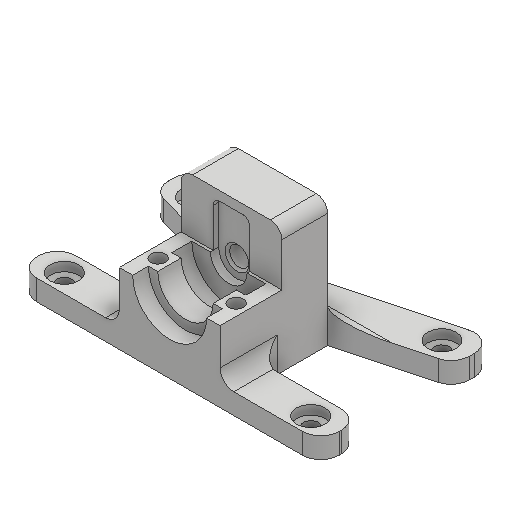
# Autodesk Inventor part: 3DP_ABS_E3DV6_Mount
Saved by Autodesk Inventor 2026.1 (Build 301233000, 233)
## iProperties
Created: 2016-01-25
Part Number: 3DP_ABS_E3DV6_Mount
Material: Ogólny
Document SubType Name: Modeling
Designer: Andrzej
Density: 1 g/cm^3
Appearance: Domyślna
Mass: 12.8574 g
Surface Area: 66.9041 cm^2
Volume: 12.8574 cm^3
Author: Andrzej
Autodesk Inventor part; units mm, degrees
ref_plane "YZ Plane" through (0, 0, 0) normal (1, 0, 0) x (0, 1, 0)
ref_plane "XZ Plane" through (0, 0, 0) normal (0, 1, 0) x (-1, 0, 0)
ref_plane "XY Plane" through (0, 0, 0) normal (0, 0, 1) x (1, 0, 0)
sketch "Szkic1" plane through (0, 0, 0) normal (0, 0, 1) x (1, 0, 0)
  line L0 (-43.0447, 20.476) -> (-43.0447, -18.4903)
  line L1 (22.9553, 20.2216) -> (22.9553, -18.4903)
  line L2 (-21.0447, 5.0097) -> (-21.0447, -9.9903)
  line L3 (0.9553, 5.0097) -> (0.9553, -9.9903)
  line L4 (-43.0447, -18.4903) -> (22.9553, -18.4903)
  line L5 (-43.0447, -9.9903) -> (-21.0447, -9.9903)
  line L6 (0.9553, -9.9903) -> (22.9553, -9.9903)
  line L7 (-21.0447, 5.0097) -> (0.9553, 5.0097)
  line L8 (-21.0447, 5.0097) -> (-43.0447, 11.1338)
  line L9 (-10.2095, 11.3357) -> (-43.0447, 20.476)
  line L10 (0.9553, 5.0097) -> (22.9553, 10.9042)
  line L11 (-10.2095, 11.3357) -> (22.9553, 20.2216)
  point P0 (0, 0)
  point P1 (-37.0447, -14.4903)
  point P2 (16.955, -14.6697)
  point P3 (-37.0447, 14.1347)
  point P4 (16.9553, 13.9553)
  dimension "d0" = 66
  dimension "d1" = 54
  dimension "d2" = 6
  dimension "d3" = 54
  dimension "d4" = 6
  dimension "d5" = 28.625
  dimension "d6" = 22
  dimension "d7" = 22
  dimension "d8" = 4
  dimension "d10" = 23.5
  dimension "d11" = 4.5
  dimension "d12" = 9
  dimension "d13" = 28.625
  dimension "d14" = 4.5
  dimension "d15" = 9
  constraints: 24 end point, 4 perpendicular, 4 point on line, 4 vertical
  measures "d0" distance between parallel lines of L1 L0
  measures "d1" distance of point (16.955, -14.67) point (-37.045, -14.49)
  measures "d2" distance from line of L0 point (-37.045, -14.49)
  measures "d3" horizontal distance of point (16.955, 13.955) point (-37.045, 14.135)
  measures "d4" distance from line of L0 point (-37.045, 14.135)
  measures "d5" distance of point (-37.045, -14.49) point (-37.045, 14.135)
  measures "d6" distance between parallel lines of L3 L2
  measures "d7" distance between parallel lines of L2 L0
  measures "d8" distance from line of L4 point (-37.045, -14.49)
  measures "d10" distance between parallel lines of L4 L7
  measures "d11" distance from line of L8 point (-37.045, 14.135)
  measures "d12" distance between parallel lines of L8 L9
  measures "d13" distance of point (16.955, -14.67) point (16.955, 13.955)
  measures "d14" distance from line of L10 point (16.955, 13.955)
  measures "d15" distance between parallel lines of L10 L11
extrude "Wyciągnięcie proste1" add sketch "Szkic1" along normal blind 4.5 contours L9 L11 L1 L10 L7 L8 L0 | L5 L2 L7 L3 L6 L1 L4 L0
hole "Otwór1" at (-37.0447, -14.4903, 0) at (16.955, -14.6697, 0) at (-37.0447, 14.1347, 0) at (16.9553, 13.9553, 0) direction (0, 0, 1) diameter 3.25 end through all
sketch "Szkic2" plane through (0, 0, 4.5) normal (0, 0, 1) x (1, 0, 0)
  line L0 (-21.0447, 5.0097) -> (-21.0447, -9.9903) projected
  line L1 (-21.0447, 5.0097) -> (0.7211, 5.0097)
  circle A0 centre (-37.0447, 14.1347) radius 1.625 projected
  circle A1 centre (-37.0447, -14.4903) radius 1.625 projected
  circle A2 centre (16.955, -14.6697) radius 1.625 projected
  circle A3 centre (16.9553, 13.9553) radius 1.625 projected
  line L2 (-43.0447, 20.476) -> (-43.0447, 11.1338) projected
  line L3 (-43.0447, 11.1338) -> (-21.0447, 5.0097) projected
  line L4 (-21.0447, 5.0097) -> (-21.0447, -9.9903) projected
  line L5 (-21.0447, -9.9903) -> (-43.0447, -9.9903) projected
  line L6 (-43.0447, -9.9903) -> (-43.0447, -18.4903) projected
  line L7 (-43.0447, -18.4903) -> (22.9553, -18.4903) projected
  line L8 (22.9553, -18.4903) -> (22.9553, -9.9903) projected
  line L9 (22.9553, -9.9903) -> (0.9553, -9.9903) projected
  line L10 (0.9553, -9.9903) -> (0.9553, 5.0097) projected
  line L11 (0.9553, 5.0097) -> (22.9553, 10.9042) projected
  line L12 (22.9553, 10.9042) -> (22.9553, 20.2216) projected
  line L13 (22.9553, 20.2216) -> (-10.2095, 11.3357) projected
  line L14 (-10.2095, 11.3357) -> (-43.0447, 20.476) projected
  line L15 (-21.0447, -4.9903) -> (0.9553, -4.9903)
  line L16 (-43.0447, -18.4903) -> (22.9553, -18.4903) projected
  line L17 (-21.0447, -4.9903) -> (0.9553, -4.9903)
  line L18 (0.9553, -4.9903) -> (0.9553, -18.4903)
  line L19 (0.9553, -18.4903) -> (-21.0447, -18.4903)
  line L20 (-21.0447, -18.4903) -> (-21.0447, -4.9903)
  line L21 (-21.0447, 5.0097) -> (0.9553, 5.0097)
  line L22 (0.9553, 5.0097) -> (0.9553, -4.9903)
  line L23 (0.9553, -4.9903) -> (-21.0447, -4.9903)
  line L24 (-21.0447, -4.9903) -> (-21.0447, 5.0097)
  circle A4 centre (-37.0447, 14.1347) radius 3.1
  circle A5 centre (16.9553, 13.9553) radius 3.1
  circle A6 centre (16.955, -14.6697) radius 3.1
  circle A7 centre (-37.0447, -14.4903) radius 3.1
  point P0 (0, 0)
  dimension "d25" = 13.5
  dimension "d31" = 6.2
  dimension "d32" = 6.2
  dimension "d33" = 6.2
  dimension "d34" = 6.2
  constraints: 20 end point, 4 centre point, 4 coincident, 4 parallel, 3 horizontal, 3 perpendicular, 3 point on line
  measures "d25" distance between parallel lines of L7 L15
  measures "d31" diameter of A4
  measures "d32" diameter of A5
  measures "d33" diameter of A6
  measures "d34" diameter of A7
extrude "Wyciągnięcie proste2" add sketch "Szkic2" along normal blind 11 contours L15 L10 L18 L7 L20 L0
extrude "Wyciągnięcie proste3" add sketch "Szkic2" along normal blind 23 contours L1 L21 L10 L15 L0
fillet "Zaokrąglenie1" radius 4 11 edges at (22.9553, 10.9042, 2.25) (22.9553, 20.2216, 2.25) (-10.2095, 11.3357, 2.25) (-43.0447, 20.476, 2.25) (-43.0447, 11.1338, 2.25) (0.9553, -9.9903, 2.25) (22.9553, -9.9903, 2.25) (22.9553, -18.4903, 2.25) (-43.0447, -18.4903, 2.25) (-43.0447, -9.9903, 2.25) (-21.0447, -9.9903, 2.25)
extrude "Wyciągnięcie proste4" cut sketch "Szkic2" against normal blind 2 contours A4 | A5 | A6 | A7
fillet "Zaokrąglenie2" radius 3 3 edges at (-10.0447, 5.0097, 4.5) (-21.0447, -12.2403, 4.5) (0.9553, -12.2403, 4.5)
fillet "Zaokrąglenie3" radius 2.5 2 edges at (-21.0447, 0.0097, 27.5) (0.9553, 0.0097, 27.5)
sketch "Szkic3" plane through (-21.0447, -18.4903, 15.5) normal (0, -1, 0) x (1, 0, 0)
  line L0 (22, 0) -> (0, 0) projected
  line L1 (0, -8) -> (0, 0) projected
  arc A0 (2.925, 0) -> (19.075, 0) centre (11, 0) ccw
  arc A1 (4.95, 0) -> (17.05, 0) centre (11, 0) ccw
  point P0 (21.0447, -15.5)
  dimension "d39" = 11
  dimension "d48" = 16.15
  dimension "d51" = 12.1
  constraints: 4 point on circle, 4 point on line, 2 centre point, 2 coincident, 1 midpoint
  measures "d39" distance from line of L1 point (11, 0)
  measures "d48" diameter of A0
  measures "d51" diameter of A1
hole "Otwór2" at (-10.0447, -18.4903, 15.5) direction (0, 1, 0) diameter 4.2 end through all
extrude "Wyciągnięcie proste5" cut sketch "Szkic3" against normal blind 12.9
extrude "Wyciągnięcie proste6" add sketch "Szkic3" against normal blind 8.55 contours A0 L0 A1
extrude "Wyciągnięcie proste7" cut sketch "Szkic3" against normal blind 3.45 contours A0 L0 A1
sketch "Szkic4" plane through (0, 0, 15.5) normal (0, 0, 1) x (1, 0, 0)
  line L0 (-3.9947, -15.0403) -> (-1.9697, -15.0403) projected
  line L1 (-3.9947, -9.9403) -> (-1.9697, -9.9403) projected
  line L2 (0.9553, -18.4903) -> (0.9553, -4.9903) projected
  line L3 (-3.9947, -15.0403) -> (-3.9947, -9.9403) projected
  line L4 (-18.1197, -9.9403) -> (-16.0947, -9.9403) projected
  line L5 (-21.0447, -4.9903) -> (-21.0447, -18.4903) projected
  point P0 (0, 0)
  point P1 (-18.5697, -12.4903)
  point P2 (-1.5197, -12.4903)
  dimension "d56" = 5.1
  dimension "d57" = 4.95
  dimension "d58" = 2.475
  dimension "d59" = 2.55
  dimension "d60" = 2.55
  dimension "d61" = 2.475
  measures "d56" distance between parallel lines of L0 L1
  measures "d57" distance between parallel lines of L2 L3
  measures "d58" distance from line of L2 point (-1.52, -12.49)
  measures "d59" distance from line of L1 point (-1.52, -12.49)
  measures "d60" distance from line of point (-18.57, -12.49) L4
  measures "d61" distance from line of point (-18.57, -12.49) L5
hole "Otwór3" at (-18.5697, -12.4903, 15.5) at (-1.5197, -12.4903, 15.5) direction (0, 0, -1) diameter 3.2 end through all
sketch "Szkic5" plane through (0, 0, 0) normal (0, 0, -1) x (-1, 0, 0)
  circle A0 centre (18.5697, -12.4903) radius 1.6 projected
  circle A1 centre (1.5197, -12.4903) radius 1.6 projected
  circle A2 centre (18.5697, -12.4903) radius 3.1
  circle A3 centre (1.5197, -12.4903) radius 3.1
  point P0 (0, 0)
  dimension "d69" = 6.2
  dimension "d70" = 6.2
  constraints: 2 centre point, 2 coincident
  measures "d69" diameter of A2
  measures "d70" diameter of A3
extrude "Wyciągnięcie proste8" cut sketch "Szkic5" against normal blind 3
sketch "Szkic6" plane through (-21.0447, -5.5903, 15.5) normal (0, -1, 0) x (1, 0, 0)
  arc A0 (7, 0) -> (15, 0) centre (11, 0) ccw
  line L0 (7, 0) -> (7, 8.5)
  line L1 (8.5, 10) -> (13.5, 10)
  line L2 (15, 8.5) -> (15, 0)
  arc A1 (8.9, 0) -> (13.1, 0) centre (11, 0) ccw projected
  arc A2 (8.5, 10) -> (7, 8.5) centre (8.5, 8.5) ccw
  arc A3 (15, 8.5) -> (13.5, 10) centre (13.5, 8.5) ccw
  point P0 (21.0447, -15.5)
  point P1 (7, 10)
  dimension "d73" = 8
  dimension "d74" = 10
  dimension "d75" = 1.5
  constraints: 6 end point, 6 point on circle, 5 tangent, 3 centre point, 2 point on line, 1 coincident, 1 equal radius, 1 horizontal, 1 perpendicular
  measures "d73" diameter of A0
  measures "d74" distance of L0.start point (7, 10)
  measures "d75" radius of A2
extrude "Wyciągnięcie proste9" cut sketch "Szkic6" against normal blind 1.8
chamfer "Faza1" distance 0.5 angle 45 2 edges at (-10.0447, 5.0097, 17.6) (-10.0447, -3.7903, 17.6)
equation "\"d13\" = d5"
equation "\"d58\" = 0.5 * d57"
equation "\"d59\" = 0.5 * d56"
equation "\"d60\" = d59"
equation "\"d61\" = d58"
equation "\"d9\" = d8"
